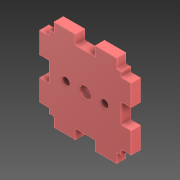
# Autodesk Inventor part: deksel lagerblok huis
Saved by Autodesk Inventor 2020 (Build 240168000, 168)
## iProperties
Created: 2020-05-19
Part Number: deksel lagerblok huis
Material: Generic
Document SubType Name: Modeling
Designer: stefa
Density: 1 g/cm^3
Appearance: Smooth - Red
Author: stefa
Autodesk Inventor part; units mm, degrees
ref_plane "YZ Plane" through (0, 0, 0) normal (1, 0, 0) x (0, 1, 0)
ref_plane "XZ Plane" through (0, 0, 0) normal (0, 1, 0) x (-1, 0, 0)
ref_plane "XY Plane" through (0, 0, 0) normal (0, 0, 1) x (1, 0, 0)
sketch "Sketch1" plane through (0, 0, 0) normal (0, 0, 1) x (1, 0, 0)
  line L0 (-47.5, -47.5) -> (47.5, -47.5)
  line L1 (47.5, -47.5) -> (47.5, 47.5)
  line L2 (47.5, 47.5) -> (-47.5, 47.5)
  line L3 (-47.5, 47.5) -> (-47.5, -47.5)
  line L4 (-47.5, -47.5) -> (47.5, 47.5) construction
  line L5 (47.5, -47.5) -> (-47.5, 47.5) construction
  line L6 (-37.5, 37.5) -> (37.5, 37.5)
  line L7 (37.5, 37.5) -> (37.5, -37.5)
  line L8 (37.5, -37.5) -> (-37.5, -37.5)
  line L9 (-37.5, -37.5) -> (-37.5, 37.5)
  line L10 (10, 47.5) -> (10, 37.5)
  line L11 (32.5, 47.5) -> (32.5, 37.5)
  line L12 (37.5, 32.5) -> (47.5, 32.5)
  line L13 (47.5, 10) -> (37.5, 10)
  line L14 (-47.5, 10) -> (-37.5, 10)
  line L15 (-47.5, 32.5) -> (-37.5, 32.5)
  line L16 (-32.5, 37.5) -> (-32.5, 47.5)
  line L17 (-10, 47.5) -> (-10, 37.5)
  line L18 (-10, -47.5) -> (-10, -37.5)
  line L19 (-32.5, -47.5) -> (-32.5, -37.5)
  line L20 (-37.5, -32.5) -> (-47.5, -32.5)
  line L21 (-47.5, -10) -> (-37.5, -10)
  line L22 (47.5, -10) -> (37.5, -10)
  line L23 (47.5, -32.5) -> (37.5, -32.5)
  line L24 (32.5, -37.5) -> (32.5, -47.5)
  line L25 (10, -47.5) -> (10, -37.5)
  circle A0 centre (0, 0) radius 6
  circle A1 centre (20, 0) radius 4
  circle A2 centre (-20, 0) radius 4
  dimension "d0" = 95
  dimension "d1" = 95
  dimension "d2" = 10
  dimension "d3" = 15
  dimension "d4" = 22.5
  dimension "d5" = 15
  dimension "d6" = 22.5
  dimension "d9" = 360
  dimension "d14" = 12
  dimension "d15" = 8
  dimension "d17" = 20
  dimension "d18" = 20
  constraints: 52 end point, 8 point on line, 6 perpendicular, 4 midpoint, 4 parallel, 3 centre point, 2 horizontal alignment, 1 coincident, 1 equal radius, 1 horizontal, 52 other
  measures "d0" distance of L2.end L1.end
  measures "d1" distance of L1.end L0.end
  measures "d2" distance between parallel lines of L2 L6
  measures "d3" distance between parallel lines of L1 L11
  measures "d4" distance between parallel lines of L11 L10
  measures "d5" distance between parallel lines of L12 L2
  measures "d6" distance between parallel lines of L13 L12
  measures "d14" diameter of A0
  measures "d15" diameter of A1
  measures "d17" distance of A0.centre A1.centre
  measures "d18" distance of point (0, 0) A2.centre
extrude "Extrusion1" add sketch "Sketch1" along normal blind 10 contours L19 L8 L18 L0 | L3 L21 L9 L20 | L8 L9 L6 L7 | L25 L8 L24 L0 | L3 L15 L9 L14 | L23 L7 L22 L1 | L2 L17 L6 L16 | L13 L7 L12 L1 | L2 L11 L6 L10
fillet "Fillet1" radius 0.5 108 edges at (10, -42.5, 10) (10, -42.5, 0) (10, -47.5, 5) (35, -37.5, 10) (35, -37.5, 0) (32.5, -37.5, 5) (32.5, -42.5, 10) (32.5, -42.5, 0) (32.5, -47.5, 5) (21.25, -47.5, 0) (21.25, -47.5, 10) (37.5, -37.5, 5) (37.5, -32.5, 5) (47.5, -21.25, 10) (47.5, -21.25, 0) (42.5, -32.5, 10) (42.5, -32.5, 0) (47.5, -32.5, 5) (37.5, -35, 0) (37.5, -35, 10) (47.5, -10, 5) (42.5, -10, 10) (37.5, 10, 5) (42.5, 10, 10) (42.5, 10, 0) (47.5, 10, 5) (37.5, -10, 5) (37.5, 0, 10) (42.5, -10, 0) (37.5, 0, 0) (32.5, 47.5, 5) (47.5, 21.25, 0) (47.5, 21.25, 10) (42.5, 32.5, 0) (47.5, 32.5, 5) (42.5, 32.5, 10) (37.5, 32.5, 5) (0, 37.5, 0) (0, 37.5, 10) (32.5, 37.5, 5) (10, 37.5, 5) (37.5, 37.5, 5) (35, 37.5, 10) (35, 37.5, 0) (37.5, 35, 0) (21.25, 47.5, 10) (10, 42.5, 10) (10, 47.5, 5) (21.25, 47.5, 0) (10, 42.5, 0) (32.5, 42.5, 10) (32.5, 42.5, 0) (37.5, 35, 10) (-10, 37.5, 5) (-10, 42.5, 10) (-10, 42.5, 0) (-10, 47.5, 5) (-21.25, 47.5, 10) (-21.25, 47.5, 0) (-32.5, 42.5, 10) (-32.5, 47.5, 5) (-32.5, 42.5, 0) (-32.5, 37.5, 5) (-37.5, 37.5, 5) (-35, 37.5, 10) (-37.5, 35, 10) (-37.5, 35, 0) (-35, 37.5, 0) (-37.5, 10, 5) (-42.5, 10, 10) (-47.5, 10, 5) (-42.5, 10, 0) (-37.5, 0, 10) (-37.5, 0, 0) (-37.5, 32.5, 5) (-42.5, 32.5, 0) (-47.5, 32.5, 5) (-47.5, 21.25, 0) (-47.5, 21.25, 10) (-42.5, 32.5, 10) (-37.5, -10, 5) (-42.5, -10, 10) (-42.5, -10, 0) (-47.5, -21.25, 10) (-47.5, -21.25, 0) (-47.5, -32.5, 5) (-42.5, -32.5, 10) (-42.5, -32.5, 0) (-37.5, -32.5, 5) (-37.5, -35, 10) (-37.5, -35, 0) (-37.5, -37.5, 5) (-35, -37.5, 10) (-35, -37.5, 0) (-47.5, -10, 5) (-32.5, -37.5, 5) (-10, -37.5, 5) (0, -37.5, 0) (10, -37.5, 5) (0, -37.5, 10) (-21.25, -47.5, 0) (-32.5, -42.5, 0) (-32.5, -47.5, 5) (-21.25, -47.5, 10) (-32.5, -42.5, 10) (-10, -47.5, 5) (-10, -42.5, 10) (-10, -42.5, 0)
equation "\"d5\" = d3"
equation "\"d6\" = d4"
equation "\"d18\" = d17"
body "Solid1"
